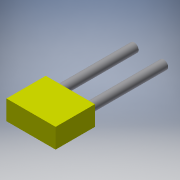
# Autodesk Inventor part: arm_safe
Saved by Autodesk Inventor 2019 (Build 230136000, 136)
## iProperties
Created: 2019-02-02
Part Number: arm_safe
Material: Generic
Document SubType Name: Modeling
Designer: suchanek
Density: 1 g/cm^3
Appearance: Default
Author: suchanek
Autodesk Inventor part; units mm, degrees
ref_plane "YZ Plane" through (0, 0, 0) normal (1, 0, 0) x (0, 1, 0)
ref_plane "XZ Plane" through (0, 0, 0) normal (0, 1, 0) x (-1, 0, 0)
ref_plane "XY Plane" through (0, 0, 0) normal (0, 0, 1) x (1, 0, 0)
sketch "Sketch1" plane through (0, 0, 0) normal (0, 0, 1) x (1, 0, 0)
  line L0 (-2.5, 7.5) -> (-27.5, 7.5)
  line L1 (-27.5, 7.5) -> (-27.5, 17.5)
  line L2 (-27.5, 17.5) -> (-2.5, 17.5)
  line L3 (-2.5, 17.5) -> (-2.5, 7.5)
  point P0 (0, 0)
  dimension "d0" = 10
  dimension "d1" = 25
  dimension "d2" = 2.5
  dimension "d3" = 7.5
  constraints: 8 end point, 2 parallel, 1 horizontal, 1 perpendicular
  measures "d0" distance of L2.end L0.start
  measures "d1" distance of L1.end L2.end
  measures "d2" distance from line of point (0, 0) L3
  measures "d3" distance from line of L0 point (0, 0)
extrude "Extrusion1" add sketch "Sketch1" along normal blind 20
sketch "Sketch2" plane through (0, 0, 20) normal (0, 0, 1) x (1, 0, 0)
  circle A0 centre (-7.5, 12.5) radius 2.25
  circle A1 centre (-22.5, 12.5) radius 2.25
  line L0 (-27.5, 7.5) -> (-2.5, 7.5) projected
  line L1 (-27.5, 17.5) -> (-27.5, 7.5) projected
  line L2 (-2.5, 7.5) -> (-2.5, 17.5) projected
  point P0 (0, 0)
  dimension "d6" = 4.5
  dimension "d7" = 5
  dimension "d8" = 5
  dimension "d9" = 5
  dimension "d10" = 5
  constraints: 2 centre point, 1 equal radius
  measures "d6" diameter of A0
  measures "d7" distance from line of L0 A0.centre
  measures "d8" distance from line of L0 A1.centre
  measures "d9" distance from line of L1 A1.centre
  measures "d10" distance from line of L2 A0.centre
extrude "Extrusion2" add sketch "Sketch2" against normal blind 60
body "Solid1"
